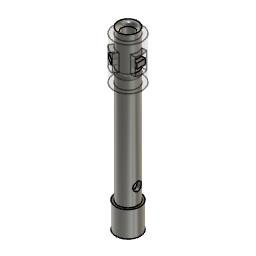
Assembly (Autodesk Fusion 360 archive; units mm, degrees)
design "RETHI Vacuum Chamber"
Autodesk Fusion 360 part; units mm, degrees
sketch "Sketch1" plane through (0, 0, 0) normal (0, 0, 1) x (1, 0, 0)
  circle A0 centre (0, 0) radius 4.445
  circle A1 centre (0, 0) radius 6.35
  circle A2 centre (0, 0) radius 2.8575
  dimension "chamberTrack" = 8.89
  dimension "d2" = 12.7
  dimension "chamberDiam" = 5.715
  constraint coincident A0.centre A1.centre
  constraint concentric A0 A2
  measures "chamberTrack" diameter of A0
  measures "d2" diameter of A1
  measures "chamberDiam" diameter of A2
extrude "Extrude1" add sketch "Sketch1" against normal blind 2.54 contours A0 makes body 1
extrude "Extrude2" add sketch "Sketch1" against normal blind 7.62 contours A1 bodies 1
extrude "Extrude3" add sketch "Sketch1" along normal blind 53.34 contours A0 bodies 1
ref_plane "WorkPlane1" through (4.445, 0, 87.4605) normal (1, 0, 0) x (0, -1, 0)
sketch "Sketch2" plane through (4.445, 0, 87.4605) normal (1, 0, 0) x (0, 1, 0)
  circle A0 centre (0, -76.2) radius 1.905
  dimension "d15" = 3.81
  measures "d15" diameter of A0
extrude "Extrude4" cut sketch "Sketch2" against normal blind 2.54 bodies 1
ref_plane "WorkPlane2" through (0, 0, 48.26) normal (0, 0, 1) x (1, 0, 0)
ref_plane "WorkPlane1" through (0, 0, 49.53) normal (0, 0, 1) x (1, 0, 0) in component "Component"
sketch "Sketch1 (2)" plane through (0, 0, 49.53) normal (0, 0, 1) x (1, 0, 0) in component "Component"
  circle A0 centre (0, 0) radius 4.445
  circle A1 centre (0, 0) radius 6.35
  circle A2 centre (0, 0) radius 4.445
  circle A3 centre (0, 0) radius 4.445
  constraint concentric A0 A2
  constraint concentric A1 A3
extrude "Extrude1'" add sketch "Sketch1 (2)" along normal blind 19.05 separate body makes body 2 in component "Component"
ref_plane "WorkPlane2" through (6.35, 0, 63.864) normal (1, 0, 0) x (0, -1, 0) in component "Component"
sketch "Sketch2 (2)" plane through (6.35, 0, 62.594) normal (1, 0, 0) x (0, 1, 0) in component "Component"
  line L0 (-2.54, 0.906) -> (2.54, 0.906)
  line L1 (2.54, 0.906) -> (2.54, -6.714)
  line L2 (2.54, -6.714) -> (-2.54, -6.714)
  line L3 (-2.54, -6.714) -> (-2.54, 0.906)
  line L4 (6.35, 5.986) -> (-6.35, 5.986)
  line L5 (6.35, -13.064) -> (-6.35, -13.064)
  dimension "compressionRoom" = 7.62
  dimension "d74" = 6.35
  constraint horizontal L0
  constraint vertical L1
  constraint horizontal L2
  constraint vertical L3
  measures "compressionRoom" distance of L0.start L2.end
  measures "d74" distance of L2 L5
extrude "Extrude2'" cut sketch "Sketch2 (2)" along normal up to surface end surface at (4.4229, -0.4426, 62.23) on bodies 2 bodies 2 in component "Component"
pattern_circular "C-Pattern1" count 3 over 360 about axis through (0, 0, 68.58) along (0, 0, -1) of 4 faces at (5.0958, 2.54, 60.96) (5.3616, 1.9489, 55.88) (5.0958, -2.54, 58.42) (5.3616, 1.9489, 63.5) on bodies 2 in component "Component"
sketch "Sketch3" plane through (0, 0, 53.34) normal (0, 0, 1) x (-1, 0, 0) in component "Component"
  circle A0 centre (0, 0) radius 2.8575
  circle A1 centre (0, 0) radius 4.445
  circle A2 centre (0, 0) radius 3.4078
  circle A3 centre (0, 0) radius 3.776
  point P0 (-0.3758, -4.4291)
  point P1 (-3.6478, -2.54)
  constraint concentric A0 A2
  constraint coincident A0.centre A1.centre
ref_plane "WorkPlane1" through (-2.6441, -4.5796, 61.595) normal (0, 0, -1) x (-0.866025, 0.5, 0) in component "Component'"
sketch "Sketch1 (3)" plane through (-2.6441, -4.5796, 61.595) normal (0, 0, -1) x (1, 0, 0) in component "Component'"
  circle A0 centre (2.6441, -4.5796) radius 2.8575
  circle A1 centre (2.6441, -4.5796) radius 4.445
  circle A2 centre (2.6441, -4.5796) radius 2.8575
  circle A3 centre (2.6441, -4.5796) radius 4.3839
  constraint concentric A0 A2
  constraint concentric A2 A3
extrude "Extrude1''" add sketch "Sketch1 (3)" against normal blind 14.605 separate body contours A3 makes body 3 in component "Component'"
ref_plane "WorkPlane2" through (4.3839, 0, 66.7779) normal (1, 0, 0) x (0, -1, 0) in component "Component'"
extrude "Extrude3'" add 1 faces at (3.8482, 0.3598, 61.595) along direction (0, 0, -1) blind 0.762 on bodies 3 bodies 3 in component "Component'"
sketch "Sketch2 (3)" plane through (4.3839, 0, 64.7583) normal (1, 0, 0) x (0, 1, 0) in component "Component'"
  line L0 (-2.032, -1.27) -> (2.032, -1.27)
  line L1 (2.032, -1.27) -> (2.032, 1.27)
  line L2 (2.032, 1.27) -> (-2.032, 1.27)
  line L3 (-2.032, 1.27) -> (-2.032, -1.27)
  dimension "d72" = 2.54
  constraint horizontal L0
  constraint vertical L1
  constraint horizontal L2
  constraint vertical L3
  measures "d72" distance of L0.end L1.end
extrude "Extrude2''" cut sketch "Sketch2 (3)" against normal blind 1.016 bodies 3 in component "Component'"
pattern_circular "C-Pattern1'" count 3 over 360 about axis through (0, 0, 76.2) along (0, 0, -1) of 4 faces at (3.7066, 0, 66.0283) (3.5401, -2.032, 64.3349) (3.5401, 2.032, 65.1816) (3.7066, 0, 63.4883) on bodies 3 in component "Component'"
sketch "Sketch1 (4)" plane through (3.3679, 0, 2.54) normal (1, 0, 0) x (0, 1, 0) in component "Component''"
  line L0 (-2.032, 66.0283) -> (-2.032, 63.4883)
  line L1 (2.032, 63.4883) -> (2.032, 66.0283)
  line L2 (2.032, 66.0283) -> (-2.032, 66.0283)
  line L3 (-1.905, 65.913) -> (1.905, 65.913)
  line L4 (1.905, 65.913) -> (1.905, 63.5918)
  line L5 (1.905, 63.5918) -> (-1.905, 63.5918)
  line L6 (-1.905, 63.5918) -> (-1.905, 65.913)
  line L7 (-2.032, 63.4883) -> (2.032, 63.4883)
  constraint horizontal L3
  constraint vertical L4
  constraint horizontal L5
  constraint vertical L6
extrude "Extrude1'''" add sketch "Sketch1 (4)" along normal blind 2.54 separate body contours L3 L4 L5 L6 makes body 4 in component "Component''"
pattern_circular "C-Pattern1''" count 3 over 360 about axis through (0, 0, 76.2) along (0, 0, -1) of bodies 4 makes body 5 at (-2.6572, -3.3324, 68.453) makes body 6 at (-3.0806, 4.0657, 68.453) in component "Component''"
fillet "Fillet1" radius 1.905 1 edges at (-2.6641, 1.0333, 76.2) on bodies 3 in component "Component'"
sketch "Sketch4" plane through (0, 0, -2.54) normal (0, 0, -1) x (1, 0, 0)
  circle A0 centre (0, 0) radius 2.8575
  circle A1 centre (0, 0) radius 4.445
  circle A2 centre (0, 0) radius 6.35
  circle A3 centre (0, 0) radius 4.445
  constraint coincident A0.centre A1.centre
  constraint concentric A2 A3
extrude "Extrude6" cut sketch "Sketch4" along normal blind 7.62 and the other way blind 2.54 contours A2 bodies 1
sketch "Sketch5" plane through (0, 0, -2.54) normal (0, 0, -1) x (1, 0, 0)
  circle A0 centre (0, 0) radius 2.8575
  circle A1 centre (0, 0) radius 4.445
  circle A2 centre (0, 0) radius 5.4229
  circle A3 centre (0, 0) radius 5.4229
  circle A4 centre (0, 0) radius 2.8575
  dimension "bearingInner" = 10.8458
  constraint coincident A0.centre A1.centre
  constraint concentric A3 A4
  measures "bearingInner" diameter of A2
extrude "Extrude7" add sketch "Sketch5" against normal blind 6.35 contours A2 A3 bodies 1
extrude "Extrude8" add 1 faces at (4.5369, 0.4114, -2.54) along direction (0, 0, -1) blind 5.08 on bodies 1 bodies 1
move_body "Move1" bodies 3 to x (1, 0, 0) y (0, 1, 0) z (0, 0, 1) at (0, 0, -7.62) in component "Component'"
move_body "Move1'" bodies 4 5 6 to x (1, 0, 0) y (0, 1, 0) z (0, 0, 1) at (0, 0, -7.62) in component "Component''"
sketch "Sketch6" plane through (0, 0, 53.34) normal (0, 0, 1) x (-1, 0, 0)
  circle A0 centre (0, 0) radius 2.8575
  circle A1 centre (0, 0) radius 4.445
  circle A2 centre (0, 0) radius 3.4737
  circle A3 centre (0, 0) radius 3.8771
  dimension "lipIn" = 6.9473
  dimension "lipOut" = 7.7543
  constraint concentric A0 A2
  constraint concentric A0 A3
  measures "lipIn" diameter of A2
  measures "lipOut" diameter of A3
extrude "Extrude9" cut sketch "Sketch6" against normal blind 1.27 contours A3 bodies 1
sketch "Sketch7" plane through (0, 0, 55.753) normal (0, 0, -1) x (1, 0, 0)
  circle A0 centre (0, 0) radius 2.8575
  circle A1 centre (0, 0) radius 4.3839
  circle A2 centre (0, 0) radius 3.4737
  circle A3 centre (0, 0) radius 3.8771
  dimension "d88" = 6.9473
  dimension "d89" = 7.7543
  constraint concentric A0 A2
  constraint coincident A0.centre A1.centre
  measures "d88" diameter of A2
  measures "d89" diameter of A3
extrude "Extrude4'" cut sketch "Sketch7" against normal blind 1.27 contours A3 sketch seen with x (1, 0, 0) y (0, 1, 0) z (0, 0, 1) at (0, 0, -2.54) bodies 3 in component "Component'"
component "Component" placed x (1, 0, 0) y (0, 1, 0) z (0, 0, 1) at (0, 0, 0)
component "Component'" placed x (1, 0, 0) y (0, 1, 0) z (0, 0, 1) at (0, 0, 2.54)
component "Component''" placed x (1, 0, 0) y (0, 1, 0) z (0, 0, 1) at (0, 0, 0)
equation "d2 = chamberTrack + 0.15 in"
equation "chamberDiam = hexDiam + 0.1 in"
equation "hexDiam = 0.125 in"
equation "length = armLength - 1.9 in"
equation "armLength = 4 in"
equation "d88 = lipIn"
equation "d89 = lipOut"

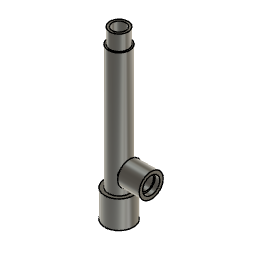
design "RETHI Vacuum Chamber Material Spring"
Autodesk Fusion 360 part; units mm, degrees
sketch "Sketch1" plane through (0, 0, 0) normal (0, 0, 1) x (1, 0, 0)
  circle A0 centre (0, 0) radius 4.445
  circle A1 centre (0, 0) radius 6.35
  circle A2 centre (0, 0) radius 2.8575
  dimension "chamberTrack" = 8.89
  dimension "d2" = 12.7
  dimension "chamberDiam" = 5.715
  constraint coincident A0.centre A1.centre
  constraint concentric A0 A2
  measures "chamberTrack" diameter of A0
  measures "d2" diameter of A1
  measures "chamberDiam" diameter of A2
extrude "Extrude1" add sketch "Sketch1" against normal blind 2.54 contours A0
extrude "Extrude2" add sketch "Sketch1" against normal blind 7.62 contours A1
extrude "Extrude3" add sketch "Sketch1" along normal blind 61.9125 contours A0
ref_plane "WorkPlane1" through (4.445, 0, 87.4605) normal (1, 0, 0) x (0, -1, 0)
sketch "Sketch2" plane through (4.445, 0, 87.4605) normal (1, 0, 0) x (0, 1, 0)
  circle A0 centre (0, -76.2) radius 1.905
  circle A1 centre (0, -76.2) radius 3.429
  dimension "d15" = 3.81
  dimension "d95" = 1.524
  measures "d15" diameter of A0
extrude "Extrude4" cut sketch "Sketch2" against normal blind 2.54 contours A0
ref_plane "WorkPlane2" through (0, 0, 56.8325) normal (0, 0, 1) x (1, 0, 0)
sketch "Sketch4" plane through (0, 0, -2.54) normal (0, 0, -1) x (1, 0, 0)
  circle A0 centre (0, 0) radius 2.8575
  circle A1 centre (0, 0) radius 4.445
  circle A2 centre (0, 0) radius 6.35
  circle A3 centre (0, 0) radius 4.445
  constraint coincident A0.centre A1.centre
  constraint concentric A2 A3
extrude "Extrude6" cut sketch "Sketch4" along normal blind 7.62 and the other way blind 2.54 contours A2
sketch "Sketch5" plane through (0, 0, -2.54) normal (0, 0, -1) x (1, 0, 0)
  circle A0 centre (0, 0) radius 2.8575
  circle A1 centre (0, 0) radius 4.445
  circle A2 centre (0, 0) radius 5.95
  circle A3 centre (0, 0) radius 5.4229
  circle A4 centre (0, 0) radius 2.8575
  dimension "bearingInner" = 11.9
  constraint coincident A0.centre A1.centre
  constraint concentric A3 A4
  measures "bearingInner" diameter of A2
extrude "Extrude7" add sketch "Sketch5" against normal blind 6.35 contours A2 | A3
extrude "Extrude8" add 1 faces at (4.8864, 0.4376, -2.54) along direction (0, 0, -1) blind 5.08
sketch "Sketch8" plane through (0, 0, 61.9125) normal (0, 0, 1) x (-1, 0, 0)
  circle A0 centre (0, 0) radius 2.8575
  circle A1 centre (0, 0) radius 4.445
  circle A2 centre (0, 0) radius 3.81
  dimension "d92" = 7.62
  constraint concentric A0 A2
  measures "d92" diameter of A2
extrude "Extrude10" cut sketch "Sketch8" against normal blind 6.35 contours A1
extrude "Extrude11" add sketch "Sketch2" along normal blind 0 and the other way blind 1.5875
sketch "Sketch9" plane through (4.445, 0, 0) normal (1, 0, 0) x (0, 1, 0)
  circle A0 centre (0, 11.2605) radius 1.905
  circle A1 centre (0, 11.2605) radius 5
  circle A2 centre (0, 11.2605) radius 1.905
  arc A3 (0, 14.6895) -> (0, 7.8315) centre (0, 11.2605) ccw
  arc A4 (0, 7.8315) -> (0, 14.6895) centre (0, 11.2605) ccw
  dimension "d100" = 10
  constraint concentric A0 A1
  constraint concentric A1 A2
  measures "d100" diameter of A1
extrude "Extrude12" add sketch "Sketch9" along normal blind 9 contours A1 | A3 A4
sketch "Sketch10" plane through (13.445, 0, 0) normal (1, 0, 0) x (0, 1, 0)
  circle A0 centre (0, 11.2605) radius 1.905
  circle A1 centre (0, 11.2605) radius 5
  circle A2 centre (0, 11.2605) radius 3.585
  circle A3 centre (0, 11.2605) radius 3
  dimension "d103" = 7.17
  dimension "d104" = 6
  constraint concentric A0 A2
  constraint concentric A2 A3
  measures "d103" diameter of A2
  measures "d104" diameter of A3
extrude "Extrude13" cut sketch "Sketch10" against normal blind 2 contours A2
extrude "Extrude14" cut 1 faces at (13.445, 2.6238, 11.1114) along direction (-1, 0, 0) blind 7.62
equation "d2 = chamberTrack + 0.15 in"
equation "chamberDiam = hexDiam + 0.1 in"
equation "hexDiam = 0.125 in"
equation "length = armLength - 1.5 in - 1.5875 mm"
equation "armLength = 4 in"
equation "compressionRoom = 0.3 in"
equation "lipIn = 0.273516 in"
equation "lipOut = 0.305287 in"
equation "d88 = lipIn"
equation "d89 = lipOut"

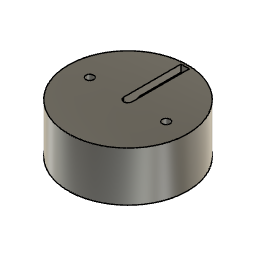
design "RETHI Hex Screwdriver Mount Cap"
Autodesk Fusion 360 part; units mm, degrees
sketch "Sketch2" plane through (0, 0, 0) normal (0, 0, 1) x (1, 0, 0)
  circle A0 centre (0, 0) radius 26.5
  dimension "diam" = 53
  constraint coincident A0.centre origin
  measures "diam" diameter of A0
extrude "Extrude1" add sketch "Sketch2" along normal blind 22 makes body 1
ref_plane "WorkPlane1" through (-26.5, 0, 42.6906) normal (-1, 0, 0) x (0, 1, 0)
ref_plane "WorkPlane2" through (0, 0, 42.6906) normal (-1, 0, 0) x (0, 1, 0)
sketch "Sketch3" plane through (0, 0, 102.2963) normal (-1, 0, 0) x (0, 1, 0)
  line L0 (0, 80.2963) -> (0, 181.8963)
  line L1 (0, 80.2963) -> (25.4, 80.2963)
  line L2 (-26.5, 80.2963) -> (26.5, 80.2963)
  line L3 (-26.5, 80.2963) -> (26.5, 80.2963)
  point P0 (0, 80.2963)
  dimension "armLength" = 101.6
  dimension "armWidth" = 25.4
  constraint vertical L0
  constraint perpendicular L0 L1
  constraint coincident P0 L0
  constraint coincident P0 L1
  constraint coincident P0 L2
  constraint midpoint P0 L3
  constraint coincident P0 L0.start
  measures "armLength" distance of P0 L0.end
  measures "armWidth" distance of P0 L1.end
ref_plane "WorkPlane6" through (0, 26.5, 5.9315) normal (0, 1, 0) x (1, 0, 0)
ref_plane "WorkPlane7" through (0, 25.4, 5.9315) normal (0, 1, 0) x (1, 0, 0)
sketch "Sketch6" plane through (0, 25.4, 14.2132) normal (0, 1, 0) x (1, 0, 0)
  line L0 (1.8331, -4.6118) -> (1.8331, -7.7868)
  line L1 (-1.8331, -7.7868) -> (-1.8331, -4.6118)
  line L2 (1.8331, -7.7868) -> (-1.8331, -7.7868)
  line L3 (-1.8331, -4.6118) -> (1.8331, -4.6118)
  point P0 (0, -7.7868)
  dimension "d187" = 3.175
  constraint vertical L0
  constraint perpendicular L1 L2
  constraint perpendicular L0 L3
  measures "d187" distance of L1.start L1.end
sketch "Sketch1" plane through (0, 0, 0) normal (0, 0, 1) x (1, 0, 0) in component "Cap"
  circle A0 centre (127, 0.0001) radius 26.5
  circle A1 centre (127, -16.9749) radius 5.125
  circle A2 centre (127, 16.9751) radius 5.125
  circle A3 centre (127, 16.9751) radius 1.7272
  circle A4 centre (127, -16.9749) radius 1.7272
  line L0 (127, -16.9749) -> (127, 16.9751)
  dimension "d69" = 53
  dimension "d81" = 10.25
  dimension "d82" = 10.25
  dimension "d85" = 33.95
  dimension "d143" = 3.4544
  dimension "d144" = 3.4544
  constraint concentric A2 A3
  constraint concentric A1 A4
  constraint coincident A1.centre A4.centre
  constraint coincident A2.centre A3.centre
  constraint vertical L0
  constraint midpoint A0.centre L0
  measures "d69" diameter of A0
  measures "d81" diameter of A1
  measures "d82" diameter of A2
  measures "d85" distance of A1.centre A2.centre
  measures "d143" diameter of A3
  measures "d144" diameter of A4
extrude "Extrude1'" add sketch "Sketch1" along normal blind 5.02 separate body contours A0 | A1 | A2 makes body 2 in component "Cap"
ref_plane "WorkPlane1" through (153.5, 0.0001, 15.298) normal (1, 0, 0) x (0, -1, 0) in component "Cap"
ref_plane "WorkPlane4" through (152.4, 0.0001, 15.298) normal (1, 0, 0) x (0, -1, 0) in component "Cap"
sketch "Sketch4" plane through (152.4, 0, 21.9945) normal (1, 0, 0) x (0, 1, 0) in component "Cap"
  line L0 (26.5001, -16.9745) -> (-26.4999, -16.9745)
  line L1 (0.0001, -16.9745) -> (0.0001, -18.562)
  line L2 (-1.833, -16.9745) -> (1.8331, -16.9745)
  line L3 (-0.9165, -18.562) -> (0.9166, -18.562)
  line L4 (0.9166, -18.562) -> (1.8331, -16.9745)
  line L5 (-1.833, -16.9745) -> (-0.9165, -18.562)
  line L6 (-1.833, -16.9745) -> (1.8331, -16.9745)
  line L7 (-18.7021, -16.9745) -> (-15.2477, -16.9745)
  line L8 (15.2479, -16.9745) -> (18.7023, -16.9745)
  dimension "d76" = 1.5875
  dimension "d77" = 120
  dimension "d78" = 120
  constraint midpoint L0 L1.start
  constraint perpendicular L0 L1
  constraint coincident L0 L2.start
  constraint coincident L0 L2.end
  constraint horizontal L3
  constraint equal L3 L5
  constraint midpoint L1.end L3
  measures "d76" distance of L1.start L1.end
  measures "d77" angle of L3 L5
  measures "d78" angle of L3 L4
sketch "Sketch7" plane through (0, 0, 22) normal (0, 0, 1) x (-1, 0, 0)
  circle A0 centre (0, 0) radius 26.5
  circle A1 centre (-16.9749, 0) radius 1.7272
  line L0 (16.9749, 0) -> (-16.9749, 0)
  circle A2 centre (16.9751, 0) radius 1.7272
  circle A3 centre (-16.9749, 0) radius 3.585
  circle A4 centre (16.9749, 0) radius 3.585
  dimension "d152" = 33.95
  dimension "d153" = 3.4544
  dimension "d154" = 3.4544
  dimension "d156" = 7.17
  dimension "d157" = 7.17
  constraint coincident A1.centre L0.end
  constraint midpoint A0.centre L0
  constraint coincident L0.start A4.centre
  measures "d152" distance of A1.centre A2.centre
  measures "d153" diameter of A1
  measures "d154" diameter of A2
  measures "d156" diameter of A3
  measures "d157" diameter of A4
extrude "Extrude3" cut sketch "Sketch7" against normal blind 8 contours A1 | A2 bodies 1
sketch "Sketch6 (2)" plane through (0, 0, 0) normal (0, 0, -1) x (1, 0, 0) in component "Cap"
  circle A0 centre (127, -0.0001) radius 26.5
  circle A1 centre (127, -0.0001) radius 8.8333
  circle A2 centre (127, 16.9749) radius 1.7272
  circle A3 centre (127, -16.9751) radius 1.7272
  circle A4 centre (127, -0.0001) radius 3
  dimension "d105" = 17.6667
  dimension "d190" = 6
  constraint concentric A0 A1
  constraint concentric A1 A4
  measures "d105" diameter of A1
  measures "d190" diameter of A4
extrude "Extrude4" add sketch "Sketch6 (2)" along normal blind 19.1861 contours A1 | A4 bodies 2 in component "Cap"
sketch "Sketch10" plane through (0, 0, 0) normal (0, 0, -1) x (1, 0, 0)
  circle A0 centre (0, 0) radius 26.5
  circle A1 centre (0, 0) radius 18.5
  dimension "bearingDiam" = 37
  constraint coincident A0.centre A1.centre
  measures "bearingDiam" diameter of A1
extrude "Extrude4'" cut sketch "Sketch10" against normal blind 12.0396 contours A1 bodies 1
extrude "Extrude9" cut sketch "Sketch6 (2)" along normal up to surface (19.1861 mm away) and the other way blind 0 contours A4 bodies 2 in component "Cap"
sketch "Sketch12" plane through (0, 0, 22) normal (0, 0, 1) x (-1, 0, 0)
  circle A0 centre (0, 0) radius 26.5
  circle A1 centre (0, 0) radius 1.8331
  circle A2 centre (-16.9749, 0) radius 1.7272
  circle A3 centre (16.9751, 0) radius 1.7272
  constraint concentric A0 A1
extrude "Extrude6" cut sketch "Sketch12" against normal up to surface (9.9604 mm away) contours A1 bodies 1
extrude "Extrude7" cut sketch "Sketch6" along normal blind 0 and the other way blind 25.5 bodies 1
move_body "Move1" bodies 2 to x (1, 0, 0) y (0, -1, 0) z (0, 0, -1) at (0, -27.5999, 38.1) in component "Cap"
move_body "Move2" bodies 2 to x (0, 1, 0) y (-1, 0, 0) z (0, 0, 1) at (-56.5474, -223.8853, -59.5692) in component "Cap"
fillet "Fillet2" radius 5 1 edges at (-32.1417, -105.1209, -21.4692) on bodies 2 in component "Cap"
ref_plane "WorkPlane6" through (-37.7808, -96.8853, 9.4824) normal (-1, 0, 0) x (0, 1, 0) in component "Cap"
sketch "Sketch12 (2)" plane through (-37.7808, -96.8853, 9.4824) normal (-1, 0, 0) x (0, 1, 0) in component "Cap"
  circle A0 centre (0, 15.3735) radius 1.25
  line L0 (0, 15.3735) -> (0, 22.2315)
  circle A1 centre (0, 22.2315) radius 1.25
  circle A2 centre (0, 22.2315) radius 3.25
  circle A3 centre (0, 15.3735) radius 3.25
  line L1 (-8.8333, 11.7655) -> (8.8333, 11.7655)
  line L2 (0, 23.4815) -> (-1.524, 23.4815)
  dimension "d196" = 2.5
  dimension "d198" = 2.5
  dimension "d207" = 6.5
  dimension "d208" = 6.5
  dimension "d218" = 13.716
  dimension "d219" = 6.858
  constraint coincident A0.centre L0.start
  constraint vertical L0
  constraint coincident L0.end A1.centre
  constraint concentric A1 A2
  constraint coincident A1 L2.start
  constraint tangent A1 L2
  constraint horizontal L2
  measures "d196" diameter of A0
  measures "d198" diameter of A1
  measures "d207" diameter of A2
  measures "d208" diameter of A3
  measures "d219" distance of A0.centre L0.end
sketch "Sketch9" plane through (0, 0, -21.4692) normal (0, 0, 1) x (-1, 0, 0) in component "Cap"
  circle A0 centre (11.9724, 96.8853) radius 1.7272
  circle A1 centre (28.9474, 96.8853) radius 26.5
  circle A2 centre (45.9224, 96.8853) radius 1.7272
  circle A3 centre (45.9224, 96.8853) radius 5.15
  circle A4 centre (11.9724, 96.8853) radius 5.15
  line L0 (45.9224, 96.8853) -> (11.9725, 96.8853)
  circle A5 centre (28.9474, 96.8853) radius 13.8333
  dimension "d145" = 10.3
  dimension "d146" = 10.3
  dimension "d147" = 33.95
  constraint coincident A2.centre A3.centre
  constraint concentric A2 A3
  measures "d145" diameter of A3
  measures "d146" diameter of A4
  measures "d147" distance of A0.centre A2.centre
extrude "Extrude10" cut sketch "Sketch12 (2)" along normal up to surface contours A0 | A1 end surface at (-31.8353, -96.0728, -8.6785) on bodies 2 bodies 2 in component "Cap"
extrude "Extrude5" [suppressed]
fillet "Fillet4" [suppressed]
extrude "Extrude11" cut sketch "Sketch12 (2)" against normal blind 1.7 draft -45 contours A0 | A1 | A2 | A3 bodies 2 in component "Cap"
sketch "Sketch13" plane through (0, 0, 18.825) normal (0, 0, 1) x (-1, 0, 0)
  line L0 (-1.8331, 0) -> (-1.8331, -25.4)
  line L1 (1.8331, -25.4) -> (1.8331, 0)
  line L2 (-1.8331, -6) -> (1.8331, -6)
  line L3 (1.8331, -6) -> (1.8331, 0)
  line L4 (1.8331, 0) -> (-1.8331, 0)
  line L5 (-1.8331, 0) -> (-1.8331, -6)
  arc A0 (-1.8331, 0) -> (1.8331, 0) centre (0, 0) ccw
  line L6 (-1.8331, -25.4) -> (1.8331, -25.4)
  dimension "d211" = 6
  constraint horizontal L2
  constraint vertical L3
  constraint horizontal L4
  constraint vertical L5
  constraint coincident L1.end L3.end
  constraint coincident L0 L2.start
  measures "d211" distance of L2.end L1.end
extrude "Extrude8" cut sketch "Sketch13" against normal blind 4 contours L0 L1 L2 L3 L5 A0 bodies 1
fillet "Fillet5" radius 1 2 edges at (0, 6, 18.825) (0, 1.8331, 14.825) on bodies 1
component "Cap" placed x (1, 0, 0) y (0, 1, 0) z (0, 0, 1) at (28.9474, 96.8853, 48.4892)
equation "d5 = ( -diam / 2 )"
equation "d12 = -( ( diam / 2 ) - 1 in )"
equation "hexDiam = 0.125 in"
equation "d69 = diam"
equation "d70 = 0.25 in - 1.33 mm"
equation "d75 = -( ( diam / 2 ) - 1 in )"
equation "d76 = hexDiam / 2"
equation "d85 = diam - 0.75 in"
equation "motorShaftDiam = 0.125 in"
equation "motorShaftLength = 0.953 in - 0.19764 in"
equation "d105 = diam / 3"
equation "d108 = motorShaftLength"
equation "chamberTrack = 0.474 in"
equation "d147 = diam - 0.75 in"
equation "d152 = diam - 0.75 in"
equation "d187 = 1.5875 * 2 mm"

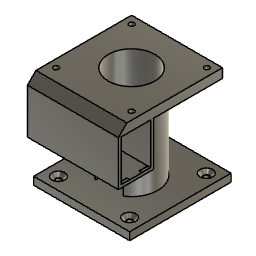
design "RETHI Screwdriver Mount"
Autodesk Fusion 360 part; units mm, degrees
sketch "Sketch1" plane through (0, 0, 0) normal (0, 0, 1) x (1, 0, 0)
  circle A0 centre (9.0475, 10.6375) radius 2.1
  circle A1 centre (44.4028, 10.6375) radius 2.1
  circle A2 centre (9.1034, 45.9928) radius 2.1
  circle A3 centre (44.4587, 45.9927) radius 2.1
  line L0 (-12.7, -12.7) -> (66.1548, -12.7)
  line L1 (66.1548, -12.7) -> (66.1548, 70.5993)
  line L2 (66.1548, 70.5993) -> (-12.7, 70.5993)
  line L3 (-12.7, 70.5993) -> (-12.7, -12.7)
  circle A4 centre (-2.54, 60.4393) radius 2.1
  circle A5 centre (55.9948, 60.4393) radius 2.1
  circle A6 centre (-2.54, -2.54) radius 2.1
  circle A7 centre (55.9948, -2.54) radius 2.1
  circle A8 centre (36.1409, 24.4553) radius 8.5
  dimension "d1" = 4.2
  dimension "d3" = 35.3553
  dimension "d8" = 35.3553
  dimension "d9" = 35.3553
  dimension "d10" = 35.3553
  dimension "d169" = 10.16
  dimension "d170" = 10.16
  dimension "d172" = 10.16
  dimension "d174" = 10.16
  dimension "d176" = 4.2
  dimension "d177" = 4.2
  dimension "d178" = 4.2
  dimension "d179" = 4.2
  dimension "d243" = 17
  constraint equal A1 A3
  constraint equal A2 A3
  constraint equal A0 A2
  constraint horizontal L0
  constraint vertical L1
  constraint horizontal L2
  constraint vertical L3
  measures "d1" diameter of A0
  measures "d3" distance of A0.centre A1.centre
  measures "d8" distance of A1.centre A3.centre
  measures "d9" distance of A0.centre A2.centre
  measures "d10" distance of A2.centre A3.centre
  measures "d169" distance of L2 A4.centre
  measures "d170" distance of L3 A4.centre
  measures "d172" distance of L1 A5.centre
  measures "d174" distance of L0 A7.centre
  measures "d176" diameter of A4
  measures "d177" diameter of A5
  measures "d178" diameter of A6
  measures "d179" diameter of A7
  measures "d243" diameter of A8
extrude "Extrude1" add sketch "Sketch1" along normal blind 6.35 contours A0 | A1 | A2 | A3 | L0 L1 L2 L3 makes body 1
sketch "Sketch2" plane through (0, 0, 6.35) normal (0, 0, 1) x (-1, 0, 0)
  circle A0 centre (-26.7268, -28.3001) radius 21.59
  circle A1 centre (-26.7268, -28.3001) radius 19.05
  line L0 (12.7, -70.5993) -> (12.7, 12.7)
  line L1 (12.7, 12.7) -> (-66.1548, 12.7)
  line L2 (-66.1548, 12.7) -> (-66.1548, -70.5993)
  line L3 (-66.1548, -70.5993) -> (12.7, -70.5993)
  circle A2 centre (-55.9948, -60.4393) radius 2.1
  circle A3 centre (2.54, 2.54) radius 2.1
  circle A4 centre (2.54, -60.4393) radius 2.1
  circle A5 centre (-55.9948, 2.54) radius 2.1
  circle A6 centre (-36.1409, -24.4553) radius 8.5
  dimension "shell" = 2.54
  dimension "d96" = 38.1
  constraint concentric A0 A1
  measures "shell" distance of A0 A1
  measures "d96" diameter of A1
extrude "Extrude7" add sketch "Sketch2" along normal blind 72.644 contours A0 bodies 1
sketch "Sketch3" plane through (0, 0, 78.994) normal (0, 0, 1) x (-1, 0, 0)
  circle A0 centre (-26.7268, -28.3001) radius 19.05
  circle A1 centre (-26.7268, -28.3001) radius 21.59
  line L0 (10.6112, -65.6381) -> (-64.0648, -65.6381)
  line L1 (-64.0648, -65.6381) -> (-64.0648, 9.0379)
  line L2 (-64.0648, 9.0379) -> (10.6112, 9.0379)
  line L3 (10.6112, 9.0379) -> (10.6112, -65.6381)
  line L4 (10.6112, -65.6381) -> (-64.0648, 9.0379)
  point P0 (-26.7268, -28.3001)
  dimension "plate" = 74.676
  constraint horizontal L0
  constraint vertical L1
  constraint horizontal L2
  constraint vertical L3
  constraint midpoint L4 P0
  constraint equal L0 L3
  measures "plate" distance of L0.start L0.end
extrude "Extrude8" add sketch "Sketch3" along normal blind 3.81 and the other way blind 3.81 contours A0 A1 L4 | A0 A1 L4 | A1 L2 L3 L4 | A1 L0 L1 L4 bodies 1
sketch "Sketch4" plane through (0, 0, 82.804) normal (0, 0, 1) x (-1, 0, 0)
  line L0 (10.6112, 9.0379) -> (-64.0648, 9.0379)
  line L1 (-64.0648, 9.0379) -> (-64.0648, -65.6381)
  line L2 (-64.0648, -65.6381) -> (10.6112, -65.6381)
  line L3 (10.6112, -65.6381) -> (10.6112, 9.0379)
  circle A0 centre (4.2612, -59.2881) radius 2.1
  circle A1 centre (-26.7268, -28.3001) radius 19.05
  circle A2 centre (-57.7148, -59.2881) radius 2.1
  circle A3 centre (4.2612, 2.6879) radius 2.1
  circle A4 centre (-57.7148, 2.6879) radius 2.1
  circle A5 centre (-42.2208, -28.3001) radius 1.5
  circle A6 centre (-34.4738, -41.7183) radius 1.5
  circle A7 centre (-18.9798, -41.7183) radius 1.5
  circle A8 centre (-11.2328, -28.3001) radius 1.5
  circle A9 centre (-18.9798, -14.8819) radius 1.5
  circle A10 centre (-34.4738, -14.8819) radius 1.5
  circle A11 centre (-26.7268, -21.1881) radius 6.35
  circle A12 centre (4.2612, 2.6879) radius 5.25
  circle A13 centre (4.2612, -59.2881) radius 5.25
  circle A14 centre (-57.7148, -59.2881) radius 5.25
  circle A15 centre (-57.7148, 2.6879) radius 5.25
  dimension "screwDiam" = 4.2
  dimension "d37" = 6.35
  dimension "d38" = 6.35
  dimension "d49" = -61.976
  dimension "d50" = 61.976
  dimension "d98" = 3
  dimension "d101" = 30.988
  dimension "d102" = 12.7
  dimension "d103" = 7.112
  dimension "d133" = -61.976
  dimension "d134" = 61.976
  dimension "d135" = 10.5
  measures "screwDiam" diameter of A0
  measures "d37" distance of L2 A0.centre
  measures "d38" distance of L3 A0.centre
  measures "d98" diameter of A5
  measures "d101" distance of A6.centre A9.centre
  measures "d102" diameter of A11
  measures "d103" vertical distance of A8.centre A11.centre
  measures "d135" diameter of A13
extrude "Extrude10" cut sketch "Sketch4" against normal up to surface (7.62 mm away) contours A0 | A2 | A3 | A4 bodies 1
sketch "Sketch2 (2)" plane through (0, 0, 82.804) normal (0, 0, 1) x (-1, 0, 0) in component "Cap"
  circle A0 centre (4.2612, -59.2881) radius 2.1
  line L0 (10.6112, 9.0379) -> (-64.0648, 9.0379)
  line L1 (-64.0648, 9.0379) -> (-64.0648, -65.6381)
  line L2 (-64.0648, -65.6381) -> (10.6112, -65.6381)
  line L3 (10.6112, -65.6381) -> (10.6112, 9.0379)
  line L4 (10.6112, -65.6381) -> (-64.0648, -65.6381)
  line L5 (-64.0648, -65.6381) -> (-64.0648, 9.0379)
  line L6 (-64.0648, 9.0379) -> (10.6112, 9.0379)
  line L7 (10.6112, 9.0379) -> (10.6112, -65.6381)
  circle A1 centre (4.2612, -59.2881) radius 2.1
  circle A2 centre (-57.7148, -59.2881) radius 2.1
  circle A3 centre (4.2612, 2.6879) radius 2.1
  circle A4 centre (-57.7148, 2.6879) radius 2.1
  circle A5 centre (-42.2208, -28.3001) radius 1.25
  circle A6 centre (-26.7268, -21.3001) radius 6.5
  circle A7 centre (-26.7268, -28.3001) radius 19.05
  circle A8 centre (-34.4738, -41.7183) radius 1.25
  circle A9 centre (-18.9798, -41.7183) radius 1.25
  circle A10 centre (-11.2328, -28.3001) radius 1.25
  circle A11 centre (-18.9798, -14.8819) radius 1.25
  circle A12 centre (-34.4738, -14.8819) radius 1.25
  circle A13 centre (4.2612, -59.2881) radius 3.585
  circle A14 centre (-57.7148, -59.2881) radius 3.585
  circle A15 centre (4.2612, 2.6879) radius 3.585
  circle A16 centre (-57.7148, 2.6879) radius 3.585
  dimension "d82" = -61.976
  dimension "d83" = 61.976
  dimension "d89" = 4.2
  dimension "d104" = 2.5
  dimension "d106" = 13
  dimension "d111" = 360
  dimension "d113" = 30.988
  dimension "d114" = 7
  dimension "d126" = 7.17
  dimension "d129" = -61.976
  dimension "d130" = 61.976
  constraint horizontal L4
  constraint vertical L5
  constraint horizontal L6
  constraint vertical L7
  constraint coincident L0.end L1.start
  constraint coincident L2.end L3.start
  constraint concentric A0 A1
  constraint concentric A1 A13
  measures "d89" diameter of A1
  measures "d104" diameter of A5
  measures "d106" diameter of A6
  measures "d113" distance of A8.centre A11.centre
  measures "d114" vertical distance of A6.centre A10.centre
  measures "d126" diameter of A13
extrude "Extrude2" add sketch "Sketch2 (2)" along normal blind 5 separate body contours L0 L1 L2 L3 L4 L5 L6 L7 | A7 | A13 | A14 | A15 | A16 makes body 2 in component "Cap"
sketch "Sketch3 (2)" plane through (0, 0, 87.804) normal (0, 0, 1) x (-1, 0, 0) in component "Cap"
  circle A0 centre (4.2612, 2.6879) radius 2.1
  circle A1 centre (4.2612, -59.2881) radius 2.1
  circle A2 centre (-18.9798, -41.7183) radius 1.25
  circle A3 centre (-57.7148, -59.2881) radius 2.1
  circle A4 centre (-34.4738, -41.7183) radius 1.25
  circle A5 centre (-26.7268, -21.3001) radius 6.5
  circle A6 centre (-42.2208, -28.3001) radius 1.25
  circle A7 centre (-57.7148, 2.6879) radius 2.1
  circle A8 centre (-11.2328, -28.3001) radius 1.25
  circle A9 centre (-18.9798, -14.8819) radius 1.25
  circle A10 centre (-34.4738, -14.8819) radius 1.25
  line L0 (10.6112, 9.0379) -> (-64.0648, 9.0379)
  line L1 (-64.0648, 9.0379) -> (-64.0648, -65.6381)
  line L2 (-64.0648, -65.6381) -> (10.6112, -65.6381)
  line L3 (10.6112, -65.6381) -> (10.6112, 9.0379)
  circle A11 centre (-42.2208, -28.3001) radius 3.25
  circle A12 centre (-26.7268, -28.3001) radius 19.05
  circle A13 centre (-34.4738, -41.7183) radius 3.25
  circle A14 centre (-18.9798, -41.7183) radius 3.25
  circle A15 centre (-11.2328, -28.3001) radius 3.25
  circle A16 centre (-18.9798, -14.8819) radius 3.25
  circle A17 centre (-34.4738, -14.8819) radius 3.25
  circle A18 centre (4.2612, -59.2881) radius 5.25
  circle A19 centre (-57.7148, -59.2881) radius 5.25
  circle A20 centre (4.2612, 2.6879) radius 5.25
  circle A21 centre (-57.7148, 2.6879) radius 5.25
  dimension "d117" = 6.5
  dimension "d119" = 360
  dimension "d158" = 10.5
  dimension "d159" = 10.5
  dimension "d160" = 10.5
  dimension "d161" = 10.5
  constraint concentric A1 A18
  constraint concentric A3 A19
  constraint concentric A0 A20
  constraint concentric A7 A21
  measures "d117" diameter of A11
  measures "d158" diameter of A18
  measures "d159" diameter of A19
  measures "d160" diameter of A20
  measures "d161" diameter of A21
extrude "Extrude3" cut sketch "Sketch3 (2)" against normal blind 1.7 draft -45 contours A2 | A4 | A6 | A8 | A9 | A10 | A11 | A13 | A14 | A15 | A16 | A17 bodies 2 in component "Cap"
sketch "Sketch10" plane through (0, 0, 6.35) normal (0, 0, 1) x (-1, 0, 0)
  circle A0 centre (-26.7268, -28.3001) radius 19.05
  circle A1 centre (-36.1409, -24.4553) radius 8.5
extrude "Extrude14" [suppressed]
sketch "Sketch11" plane through (0, 0, 6.35) normal (0, 0, 1) x (-1, 0, 0)
  circle A0 centre (-26.7268, -28.3001) radius 21.59
  circle A1 centre (-9.0475, -10.6375) radius 3.585
  circle A2 centre (-44.4028, -10.6375) radius 3.585
  circle A3 centre (-9.1034, -45.9928) radius 3.585
  circle A4 centre (-44.4587, -45.9927) radius 3.585
  line L0 (12.7, -70.5993) -> (12.7, 12.7)
  line L1 (12.7, 12.7) -> (-66.1548, 12.7)
  line L2 (-66.1548, 12.7) -> (-66.1548, -70.5993)
  line L3 (-66.1548, -70.5993) -> (12.7, -70.5993)
  circle A5 centre (-55.9948, 2.54) radius 2.1
  circle A6 centre (2.54, -60.4393) radius 2.1
  circle A7 centre (2.54, 2.54) radius 2.1
  circle A8 centre (-55.9948, -60.4393) radius 2.1
  dimension "d138" = 7.17
  dimension "d139" = 7.17
  dimension "d140" = 7.17
  dimension "d141" = 7.17
  measures "d138" diameter of A1
  measures "d139" diameter of A2
  measures "d140" diameter of A3
  measures "d141" diameter of A4
sketch "Sketch1 (2)" plane through (0, 0, 0) normal (0, 0, 1) x (1, 0, 0) in component "Connector"
  line L0 (-12.7, -12.7) -> (66.1548, -12.7)
  line L1 (66.1548, -12.7) -> (66.1548, 70.5993)
  line L2 (66.1548, 70.5993) -> (-12.7, 70.5993)
  line L3 (-12.7, 70.5993) -> (-12.7, -12.7)
  circle A0 centre (55.9948, -2.54) radius 2.1
  circle A1 centre (-2.54, -2.54) radius 2.1
  circle A2 centre (9.1034, 10.6375) radius 2.1
  circle A3 centre (44.4587, 10.6375) radius 2.1
  circle A4 centre (44.4587, 45.9928) radius 2.1
  circle A5 centre (9.1034, 45.9928) radius 2.1
  circle A6 centre (-2.54, 60.4393) radius 2.1
  circle A7 centre (55.9948, 60.4393) radius 2.1
  circle A8 centre (9.1034, 45.9928) radius 5.25
  circle A9 centre (44.4587, 45.9928) radius 5.25
  circle A10 centre (9.1034, 10.6375) radius 5.25
  circle A11 centre (44.4587, 10.6375) radius 5.25
  circle A12 centre (-2.54, -2.54) radius 3.585
  circle A13 centre (55.9948, -2.54) radius 3.585
  circle A14 centre (-2.54, 60.4393) radius 3.585
  circle A15 centre (55.9948, 60.4393) radius 3.585
  circle A16 centre (36.1409, 24.4553) radius 8.5
  dimension "d148" = 4.2
  dimension "d149" = 10.16
  dimension "d150" = 4.2
  dimension "d151" = 4.2
  dimension "d152" = 4.2
  dimension "d153" = 4.2
  dimension "d154" = 4.2
  dimension "d155" = 4.2
  dimension "d156" = 10.16
  dimension "d157" = 4.2
  dimension "d186" = 10.5
  dimension "d187" = 10.5
  dimension "d188" = 10.5
  dimension "d189" = 10.5
  dimension "d194" = 7.17
  dimension "d195" = 7.17
  dimension "d196" = 7.17
  dimension "d197" = 7.17
  dimension "d202" = 17
  constraint horizontal L0
  constraint vertical L1
  constraint horizontal L2
  constraint vertical L3
  constraint concentric A5 A8
  constraint concentric A4 A9
  constraint concentric A2 A10
  constraint concentric A3 A11
  constraint concentric A1 A12
  constraint concentric A0 A13
  constraint concentric A6 A14
  constraint concentric A7 A15
  measures "d148" diameter of A0
  measures "d149" distance of L1 A0.centre
  measures "d150" diameter of A1
  measures "d151" diameter of A2
  measures "d152" diameter of A3
  measures "d153" diameter of A4
  measures "d154" diameter of A5
  measures "d155" diameter of A6
  measures "d156" distance of L2 A6.centre
  measures "d157" diameter of A7
  measures "d186" diameter of A8
  measures "d187" diameter of A9
  measures "d188" diameter of A10
  measures "d189" diameter of A11
  measures "d194" diameter of A12
  measures "d195" diameter of A13
  measures "d196" diameter of A14
  measures "d197" diameter of A15
  measures "d202" diameter of A16
extrude "Extrude4" cut sketch "Sketch3 (2)" against normal blind 2.8 draft -45 contours A0 | A1 | A3 | A7 | A18 | A19 | A20 | A21 bodies 2 in component "Cap"
sketch "Sketch12" plane through (0, 0, 6.35) normal (0, 0, 1) x (-1, 0, 0)
  line L0 (12.7, -70.5993) -> (12.7, 12.7)
  line L1 (12.7, 12.7) -> (-66.1548, 12.7)
  line L2 (-66.1548, 12.7) -> (-66.1548, -70.5993)
  line L3 (-66.1548, -70.5993) -> (12.7, -70.5993)
  circle A0 centre (2.54, 2.54) radius 2.1
  circle A1 centre (-55.9948, -60.4393) radius 2.1
  circle A2 centre (-55.9948, 2.54) radius 2.1
  circle A3 centre (2.54, -60.4393) radius 2.1
  circle A4 centre (-26.7268, -28.3001) radius 21.59
  circle A5 centre (2.54, -60.4393) radius 5.25
  circle A6 centre (-55.9948, -60.4393) radius 5.25
  circle A7 centre (2.54, 2.54) radius 5.25
  circle A8 centre (-55.9948, 2.54) radius 5.25
  dimension "d180" = 10.5
  dimension "d181" = 10.5
  dimension "d182" = 10.5
  dimension "d183" = 10.5
  constraint concentric A3 A5
  constraint concentric A1 A6
  constraint concentric A0 A7
  constraint concentric A2 A8
  measures "d180" diameter of A5
  measures "d181" diameter of A6
  measures "d182" diameter of A7
  measures "d183" diameter of A8
extrude "Extrude16" cut sketch "Sketch12" against normal blind 2.8 draft -45 contours A0 | A1 | A2 | A3 | A5 | A6 | A7 | A8 bodies 1
extrude "Extrude1'" add sketch "Sketch1 (2)" against normal blind 6.35 separate body contours L0 L1 L2 L3 | A8 | A9 | A10 | A11 | A12 | A13 | A14 | A15 makes body 3 in component "Connector"
extrude "Extrude2'" cut sketch "Sketch1 (2)" against normal blind 3 draft -46 contours A2 | A3 | A4 | A5 | A8 | A9 | A10 | A11 bodies 3 in component "Connector"
extrude "Extrude3'" [suppressed] in component "Connector"
ref_plane "WorkPlane3" through (26.7268, 6.7101, 16.7907) normal (0, -1, 0) x (-1, 0, 0)
sketch "Sketch14" plane through (26.7268, 6.7101, 16.7907) normal (0, -1, 0) x (-1, 0, 0)
  line L0 (-11.43, 10.4407) -> (-11.43, 0.2807)
  line L1 (-11.43, 0.2807) -> (11.43, 0.2807)
  line L2 (11.43, 0.2807) -> (11.43, 10.4407)
  line L3 (11.43, 10.4407) -> (-11.43, 10.4407)
  line L4 (21.59, 10.4407) -> (-21.59, 10.4407)
  dimension "d215" = 22.86
  dimension "d216" = 10.16
  constraint horizontal L3
  constraint vertical L0
  constraint horizontal L1
  constraint vertical L2
  constraint midpoint L3 L4
  measures "d215" distance of L2.end L0.start
  measures "d216" distance of L1.end L2.end
extrude "Extrude18" cut sketch "Sketch14" along normal blind 4 and the other way blind 6 bodies 1
sketch "Sketch15" plane through (0, 0, 6.35) normal (0, 0, 1) x (-1, 0, 0)
  circle A0 centre (-55.9948, 2.54) radius 5.25
  circle A1 centre (2.54, -60.4393) radius 5.25
  circle A2 centre (2.54, 2.54) radius 5.25
  circle A3 centre (-55.9948, -60.4393) radius 5.25
  line L0 (12.7, -70.5993) -> (12.7, 12.7)
  line L1 (12.7, 12.7) -> (-66.1548, 12.7)
  line L2 (-66.1548, 12.7) -> (-66.1548, -70.5993)
  line L3 (-66.1548, -70.5993) -> (12.7, -70.5993)
  arc A4 (-37.6746, -12.7101) -> (-15.779, -12.7101) centre (-26.7268, -28.3001) ccw
  line L4 (-15.2968, -12.7101) -> (-15.2968, -9.9839)
  arc A5 (-38.1568, -9.9839) -> (-15.2968, -9.9839) centre (-26.7268, -28.3001) ccw
  line L5 (-38.1568, -9.9839) -> (-38.1568, -12.7101)
  circle A6 centre (-36.1409, -24.4553) radius 8.5
  line L6 (-15.779, -12.7101) -> (-15.2968, -12.7101)
  line L7 (-38.1568, -12.7101) -> (-37.6746, -12.7101)
sketch "Sketch16" plane through (0, 0, 75.184) normal (0, 0, -1) x (1, 0, 0)
  circle A0 centre (57.7148, -59.2881) radius 2.1
  circle A1 centre (57.7148, 2.6879) radius 2.1
  circle A2 centre (-4.2612, -59.2881) radius 2.1
  circle A3 centre (-4.2612, 2.6879) radius 2.1
  line L0 (64.0648, 9.0379) -> (-10.6112, 9.0379)
  line L1 (-10.6112, 9.0379) -> (-10.6112, -65.6381)
  line L2 (-10.6112, -65.6381) -> (64.0648, -65.6381)
  line L3 (64.0648, -65.6381) -> (64.0648, 9.0379)
  circle A4 centre (26.7268, -28.3001) radius 21.59
  line L4 (61.7268, -6.7101) -> (-8.2732, -6.7101)
  line L5 (-8.2732, -6.7101) -> (-8.2732, 17.5399)
  line L6 (-8.2732, 17.5399) -> (61.7268, 17.5399)
  line L7 (61.7268, 17.5399) -> (61.7268, -6.7101)
  line L8 (-10.6112, -9.0481) -> (-10.6112, 19.8779)
  line L9 (-10.6112, 19.8779) -> (64.0648, 19.8779)
  line L10 (64.0648, 19.8779) -> (64.0648, -9.0481)
  line L11 (64.0648, -9.0481) -> (36.4986, -9.0481)
  line L12 (16.9549, -9.0481) -> (-10.6112, -9.0481)
  arc A5 (36.4986, -9.0481) -> (16.9549, -9.0481) centre (26.7268, -28.3001) ccw
  dimension "d223" = 24.25
  dimension "d224" = 70
  constraint horizontal L4
  constraint tangent A4 L4
  constraint perpendicular L0 L5
  constraint perpendicular L5 L6
  constraint perpendicular L4 L7
  constraint coincident A4 L11.end
  constraint coincident A4 L12.start
  constraint collinear L11 L12
  constraint concentric A4 A5
  constraint tangent L4 A5
  measures "d223" distance of L4.end L5.end
  measures "d224" distance of L5.end L6.end
extrude "Extrude19" add sketch "Sketch16" along normal blind 34 contours L0 L3 A4 L4 L7 L10 L11 A5 | L0 L5 L6 L7 L8 L9 L10 | L0 L1 A4 L4 L5 L8 L12 A5 bodies 1
sketch "Sketch17" plane through (0, 0, 41.184) normal (0, 0, -1) x (1, 0, 0)
  arc A0 (26.7268, -6.7101) -> (16.9549, -9.0481) centre (26.7268, -28.3001) ccw
  line L0 (26.7268, -6.7101) -> (-8.2732, -6.7101)
  line L1 (-8.2732, -6.7101) -> (-8.2732, 17.5399)
  line L2 (-8.2732, 17.5399) -> (61.7268, 17.5399)
  line L3 (61.7268, 17.5399) -> (61.7268, -6.7101)
  line L4 (61.7268, -6.7101) -> (26.7268, -6.7101)
  arc A1 (36.4986, -9.0481) -> (26.7268, -6.7101) centre (26.7268, -28.3001) ccw
  line L5 (36.4986, -9.0481) -> (64.0648, -9.0481)
  line L6 (64.0648, -9.0481) -> (64.0648, 19.8779)
  line L7 (64.0648, 19.8779) -> (-10.6112, 19.8779)
  line L8 (-10.6112, 19.8779) -> (-10.6112, -9.0481)
  line L9 (-10.6112, -9.0481) -> (16.9549, -9.0481)
  line L10 (-10.6112, 19.8779) -> (64.0648, 19.8779)
  line L11 (64.0648, 19.8779) -> (64.0648, -9.0481)
  line L12 (64.0648, -9.0481) -> (-10.6112, -9.0481)
  line L13 (-10.6112, -9.0481) -> (-10.6112, 19.8779)
  constraint horizontal L10
  constraint vertical L11
  constraint horizontal L12
  constraint vertical L13
  constraint coincident L5.end L6.start
  constraint coincident L7.end L8.start
extrude "Extrude20" add sketch "Sketch17" along normal blind 2.338 contours L0 L1 L2 L3 L4 | A0 A1 L5 L6 L7 L8 L9 L10 L11 L12 L13 bodies 1
sketch "Sketch18" plane through (0, -9.0379, 0) normal (0, -1, 0) x (1, 0, 0)
  line L0 (64.0648, 75.184) -> (64.0648, 82.804)
  line L1 (64.0648, 82.804) -> (-10.6112, 82.804)
  line L2 (-10.6112, 82.804) -> (-10.6112, 75.184)
  line L3 (-10.6112, 75.184) -> (-8.2732, 75.184)
  line L4 (-8.2732, 75.184) -> (61.7268, 75.184)
  line L5 (61.7268, 75.184) -> (64.0648, 75.184)
  line L6 (-10.6112, 75.184) -> (64.0648, 75.184)
  line L7 (64.0648, 75.184) -> (64.0648, 82.804)
  line L8 (64.0648, 82.804) -> (-10.6112, 82.804)
  line L9 (-10.6112, 82.804) -> (-10.6112, 75.184)
  constraint horizontal L6
  constraint vertical L7
  constraint horizontal L8
  constraint vertical L9
  constraint coincident L2.end L3.start
  constraint coincident L1.end L8
extrude "Extrude21" add sketch "Sketch18" along normal up to surface (10.84 mm away) bodies 1
sketch "Sketch19" plane through (-10.6112, 0, 0) normal (-1, 0, 0) x (0, -1, 0)
  line L0 (19.8779, 82.804) -> (-65.6381, 82.804)
  line L1 (-65.6381, 82.804) -> (-65.6381, 75.184)
  line L2 (-65.6381, 75.184) -> (-9.0481, 75.184)
  line L3 (-9.0481, 75.184) -> (-9.0481, 38.846)
  line L4 (-9.0481, 38.846) -> (19.8779, 38.846)
  line L5 (19.8779, 38.846) -> (19.8779, 82.804)
  line L6 (0.4149, 75.184) -> (10.4149, 75.184)
  line L7 (10.4149, 75.184) -> (10.4149, 41.184)
  line L8 (10.4149, 41.184) -> (0.4149, 41.184)
  line L9 (0.4149, 41.184) -> (0.4149, 75.184)
  dimension "d233" = 10
  dimension "d234" = 34
  dimension "d245" = 7.62
  constraint horizontal L6
  constraint vertical L7
  constraint horizontal L8
  constraint vertical L9
  measures "d233" distance of L6.start L6.end
  measures "d234" distance of L6.start L8.end
  measures "d245" distance of L0 L6
extrude "Extrude22" cut sketch "Sketch19" against normal blind 95 contours L6 L7 L8 L9 bodies 1
sketch "Sketch20" plane through (64.0648, 0, 0) normal (1, 0, 0) x (0, 1, 0)
  line L0 (-10.4149, 41.184) -> (-10.4149, 75.184)
  line L1 (-10.4149, 75.184) -> (-0.4149, 75.184)
  line L2 (-0.4149, 75.184) -> (-0.4149, 41.184)
  line L3 (-0.4149, 41.184) -> (-10.4149, 41.184)
  line L4 (65.6381, 75.184) -> (65.6381, 82.804)
  line L5 (65.6381, 82.804) -> (-19.8779, 82.804)
  line L6 (-19.8779, 82.804) -> (-19.8779, 38.846)
  line L7 (-19.8779, 38.846) -> (9.0481, 38.846)
  line L8 (9.0481, 38.846) -> (9.0481, 75.184)
  line L9 (9.0481, 75.184) -> (65.6381, 75.184)
  line L10 (-17.5399, 75.184) -> (6.7101, 75.184)
  line L11 (6.7101, 75.184) -> (6.7101, 41.35)
  line L12 (6.7101, 41.35) -> (-17.5399, 41.35)
  line L13 (-17.5399, 41.35) -> (-17.5399, 75.184)
  dimension "d238" = 2.338
  dimension "d239" = 2.338
  dimension "d246" = 7.62
  dimension "d247" = 2.504
  constraint horizontal L10
  constraint vertical L11
  constraint horizontal L12
  constraint vertical L13
  measures "d238" distance of L6 L13
  measures "d239" distance of L8 L11
  measures "d246" distance of L5 L10
  measures "d247" distance of L7 L12
extrude "Extrude23" cut sketch "Sketch20" against normal blind 10 contours L0 L10 L12 L13 | L2 L10 L11 L12 bodies 1
chamfer "Chamfer1" distance 7 angle 45 1 edges at (26.7268, -19.8779, 82.804) on bodies 1
component "Cap" placed x (1, 0, 0) y (0, 1, 0) z (0, 0, 1) at (0, 0, 0)
component "Connector" placed x (1, 0, 0) y (0, 1, 0) z (0, 0, 1) at (0, 0, 0)
equation "d1 = screwDiam"
equation "wiresDiam = 0.141205 in"
equation "motorDiam = 1.47 in"
equation "motorShaftLength = 0.5 in"
equation "motorLength = 2.86 in"
equation "shaftDiam = 0.1 in"
equation "plate = motorDiam * 2"
equation "d49 = -plate + 0.5 in"
equation "d50 = plate - 0.5 in"
equation "motorShaftDiam = 0.25 in"
equation "d82 = -plate + 0.5 in"
equation "d83 = plate - 0.5 in"
equation "d89 = screwDiam"
equation "d102 = motorShaftDiam * 2"
equation "d129 = -plate + 0.5 in"
equation "d130 = plate - 0.5 in"
equation "d148 = screwDiam"
equation "d150 = screwDiam"
equation "d151 = screwDiam"
equation "d152 = screwDiam"
equation "d153 = screwDiam"
equation "d154 = screwDiam"
equation "d155 = screwDiam"
equation "d157 = screwDiam"
equation "d176 = screwDiam"
equation "d177 = screwDiam"
equation "d178 = screwDiam"
equation "d179 = screwDiam"
